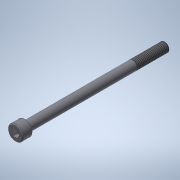
# Autodesk Inventor part: SCREW,SOCKET HD,P,12.9,M8X1.25X120MM
Saved by Autodesk Inventor 2022.4 (Build 264492000, 492)
## iProperties
Category: _
Manager: 100-28226
Created: 2022-09-14
Part Number: SCREW,SOCKET HD,P,12.9,M8X1.25X120MM
Checked By: 0003694547
Engr Approved By: P
User Status: Released
Material: Steel, MS
Description: SCREW,SOCKET HD,P,12.9,M8X1.25X120MM
Document SubType Name: Modeling
Mfg Approved By: Bill.Nguyen
Designer: Clint.Matte
Manufacturer: Standard
Standards Organization: Custom
Density: 7.86 g/cm^3
Appearance: Metal-Steel
Mass: 54.6626 g
Surface Area: 36.6519 cm^2
Volume: 6.95453 cm^3
CN_MASS: 0.05
CN_SERVICEABLE: _
FIRST_DESCRIPTION: M8X1.25X120MM
SECOND_DESCRIPTION: WV
THIRD_DESCRIPTION: _
ModelCat: Uncategorized
PTC_WM_ITERATION: 2
PTC_WM_ORGANIZATION_ID: CLWC
PTC_WM_LIFECYCLE: CLWC_CAD_LC
Subject: FMPSHMA080125120
Author: -
Keywords: DEFAULT
Revision Number: IR
Autodesk Inventor part; units mm, degrees
ref_plane "YZ Plane" through (0, 0, 0) normal (1, 0, 0) x (0, 1, 0)
ref_plane "XZ Plane" through (0, 0, 0) normal (0, 1, 0) x (-1, 0, 0)
ref_plane "XY Plane" through (0, 0, 0) normal (0, 0, 1) x (1, 0, 0)
sketch "Sketch3" plane through (0, 0, 0) normal (0, 0, 1) x (1, 0, 0)
  circle A0 centre (0, 0) radius 4
  dimension "Diameter" = 8
  constraints: 1 centre point, 1 coincident
  measures "Diameter" diameter of A0
extrude "Extrusion1" add sketch "Sketch3" against normal blind 120
sketch "Sketch4" plane through (0, 0, 0) normal (0, 0, 1) x (1, 0, 0)
  circle A0 centre (0, 0) radius 4 projected
  circle A1 centre (0, 0) radius 6.5
  dimension "Head_Diameter" = 13
  constraints: 1 centre point, 1 coincident
  measures "Head_Diameter" diameter of A1
extrude "Extrusion2" add sketch "Sketch4" along normal blind 8 contours A0 | A1
sketch "Sketch5" plane through (0, 0, 8) normal (0, 0, 1) x (1, 0, 0)
  circle A0 centre (0, 0) radius 6.5 projected
  line L0 (3.4641, 0) -> (1.7321, -3)
  line L1 (1.7321, -3) -> (-1.7321, -3)
  line L2 (-1.7321, -3) -> (-3.4641, 0)
  line L3 (-3.4641, 0) -> (-1.7321, 3)
  line L4 (-1.7321, 3) -> (1.7321, 3)
  line L5 (1.7321, 3) -> (3.4641, 0)
  line L6 (0, 0) -> (3.4641, 0) construction
  dimension "Hex_Width" = 6
  constraints: 14 end point, 1 coincident, 1 horizontal, 13 other
  measures "Hex_Width" distance between parallel lines of L1 L4
extrude "Extrusion3" cut sketch "Sketch5" against normal blind 4 contours L0 L1 L2 L3 L4 L5
thread "Thread1" size "M8x1.25" class "4g6g" standard "ANSI Metric M Profile" length 28
chamfer "Chamfer1" distance 0.8 angle 45 1 edges at (-6.5, 0, 8)
chamfer "Chamfer2" distance 0.4 angle 45 1 edges at (-4, 0, -120)
equation "\"d14\" = 0.5 * Chamfer"
equation "\"Chamfer\" = 0.8"
body "Solid1"
